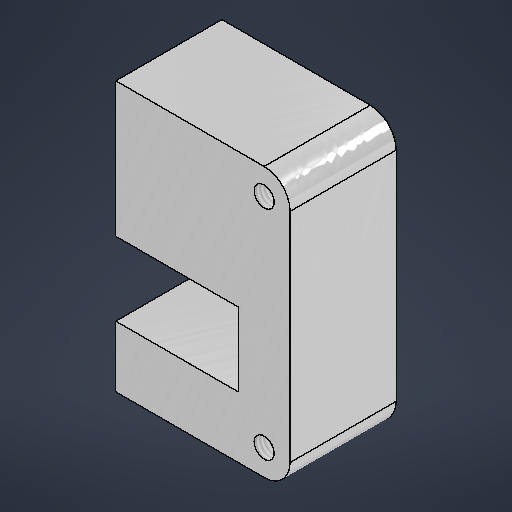
# Autodesk Inventor part: A Idler
Saved by Autodesk Inventor 2026 (Build 300175050, 175E)
## iProperties
Created: 2025-04-15
Part Number: A Idler
Material: Aluminum 6061
Document SubType Name: Modeling
Designer: Joshua Eah
Density: 2.7 g/cm^3
Appearance: Machined - Aluminum
Author: Joshua Eah
Autodesk Inventor part; units mm, degrees
ref_plane "YZ Plane" through (0, 0, 0) normal (1, 0, 0) x (0, 1, 0)
ref_plane "XZ Plane" through (0, 0, 0) normal (0, 1, 0) x (-1, 0, 0)
ref_plane "XY Plane" through (0, 0, 0) normal (0, 0, 1) x (1, 0, 0)
sketch "Base Profile" plane through (0, 0, 0) normal (0, 1, 0) x (-1, 0, 0)
  line L0 (0, 0) -> (13, 0)
  line L1 (13, 0) -> (13, -21.35)
  line L2 (13, -21.35) -> (0, -21.35)
  line L3 (0, -21.35) -> (0, 0)
  dimension "d407" = 13
  dimension "d408" = 21.35
  constraints: 8 end point, 2 parallel, 1 horizontal, 1 perpendicular
  measures "d407" distance of L1.end L2.end
  measures "d408" distance of L0.end L1.end
extrude "Extrusion21" add sketch "Base Profile" along normal blind 33
sketch "Front Profile" plane through (0, 0, 0) normal (1, 0, 0) x (0, 0, -1)
  line L0 (0, 0) -> (21.35, 0) projected
  line L1 (21.35, 0) -> (21.35, 33) projected
  line L2 (0, 33) -> (21.35, 33) projected
  line L3 (0, 0) -> (0, 33) projected
  line L4 (0, 0) -> (0, 33) projected
  line L5 (0, 16.5) -> (15, 16.5)
  line L6 (15, 16.5) -> (15, 7.5)
  line L7 (15, 7.5) -> (0, 7.5)
  line L8 (0, 7.5) -> (0, 16.5)
  line L9 (15, 33) -> (15, 0)
  line L10 (21.35, 0) -> (21.35, 33) projected
  line L11 (21.35, 16.5) -> (15, 16.5) construction
  circle A0 centre (18.175, 29.825) radius 3.175
  circle A1 centre (18.175, 3.175) radius 3.175
  point P0 (0, 7.5)
  point P1 (18.175, 16.5)
  dimension "d411" = 6.35
  dimension "d412" = 7.5
  dimension "d413" = 9
  constraints: 12 end point, 5 midpoint, 2 centre point, 2 parallel, 2 perpendicular, 2 point on line, 2 tangent, 1 horizontal, 1 symmetric about line, 1 vertical alignment, 1 other
  measures "d411" distance between parallel lines of L1 L6
  measures "d412" distance between parallel lines of L0 L7
  measures "d413" distance between parallel lines of L5 L7
extrude "Extrusion22" cut sketch "Front Profile" against normal through all contours L3 L5 L6 L7
hole "Hole27" at (0, 29.825, -18.175) at (0, 3.175, -18.175) direction (-1, 0, 0) diameter 2.459 end through all thread size "M3x0.5" class "6H" standard "ANSI Metric M Profile"
fillet "Fillet4" radius 3.175 2 edges at (-6.5, 33, -21.35) (-6.5, 0, -21.35)
equation "\"extrusionWidth\" = 15"
equation "\"bearingOffsetFromBottom\" = 7.5"
equation "\"extrusionOffset\" = 33"
equation "\"bearingStackHeight\" = 9"
equation "\"bearingSlotLength\" = 5"
equation "\"bearingClearance\" = 13"
body "Solid3"
